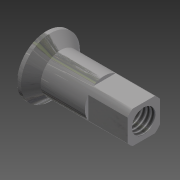
# Autodesk Inventor part: Nypel_szprychy
Saved by Autodesk Inventor 2015 (Build 190159000, 159)
## iProperties
Created: 2015-11-24
Part Number: Nypel_szprychy
Material: Stal nierdzewna
Document SubType Name: Modeling
Designer: graaapsik
Density: 8.08 g/cm^3
Appearance: Częściowo polerowany
Author: graaapsik
Autodesk Inventor part; units mm, degrees
ref_plane "YZ Plane" through (0, 0, 0) normal (1, 0, 0) x (0, 1, 0)
ref_plane "XZ Plane" through (0, 0, 0) normal (0, 1, 0) x (-1, 0, 0)
ref_plane "XY Plane" through (0, 0, 0) normal (0, 0, 1) x (1, 0, 0)
sketch "Szkic1" plane through (0, 0, 0) normal (0, 0, 1) x (1, 0, 0)
  line L0 (9.9, 0) -> (9.9, 2)
  line L1 (9.9, 2) -> (1.4, 2)
  line L2 (1.4, 2) -> (0.4, 3)
  line L3 (0.4, 3) -> (0, 3)
  arc A0 (0, 3) -> (-1.4487, 0) centre (8.1549, -2.7877) ccw
  line L4 (-1.1, 1) -> (9.9, 1) construction
  line L5 (-1.4487, 0) -> (0, 0)
  line L6 (9.9, 0) -> (0, 0)
  dimension "d1" = 11
  dimension "d2" = 1.1
  dimension "d3" = 10
  dimension "d9" = 2.5
  dimension "d10" = 45
  dimension "d11" = 1
  dimension "d12" = 3
  constraints: 14 end point, 5 point on circle, 3 horizontal, 1 centre point, 1 coincident, 1 collinear, 1 midpoint, 1 parallel, 1 vertical, 1 vertical alignment
  measures "d1" distance from line of L0 L4.start
  measures "d2" horizontal distance of L3.end L4.start
  measures "d3" radius of A0
  measures "d9" horizontal distance of L1.end L4.start
  measures "d10" angle of L4 L2
  measures "d11" distance between parallel lines of L6 L4
  measures "d12" distance between parallel lines of L3 L6
revolve "Obrót1" add sketch "Szkic1" angle 360 about axis through (9.9, 0, 0) along (-1, 0, 0)
sketch "Szkic2" plane through (9.9, 0, 0) normal (1, 0, 0) x (0, 0, -1)
  circle A0 centre (0, 0) radius 2 projected
  line L0 (-1.1303, -1.65) -> (1.1303, -1.65)
  line L1 (1.65, -1.1303) -> (1.65, 1.1303)
  line L2 (1.1303, 1.65) -> (-1.1303, 1.65)
  line L3 (-1.65, 1.1303) -> (-1.65, -1.1303)
  line L4 (-1.65, -1.65) -> (1.65, 1.65) construction
  line L5 (1.65, -1.65) -> (-1.65, 1.65) construction
  dimension "d14" = 3.3
  dimension "d15" = 3.3
  constraints: 12 end point, 2 midpoint, 2 parallel, 1 horizontal, 1 perpendicular, 9 other
  measures "d14" distance of L5.end L4.end
  measures "d15" distance of L5.start L4.end
extrude "Wyciągnięcie proste2" cut sketch "Szkic2" against normal blind 4 contours A0 L1 | L2 A0 | A0 L0 | L3 A0
sketch "Szkic3" plane through (9.9, -1.1303, -1.65) normal (1, 0, 0) x (0, 0, -1)
  line L0 (-2.7803, -0.5197) -> (-0.5197, -0.5197) projected
  arc A0 (-0.5197, -0.5197) -> (0, 0) centre (-1.65, 1.1303) ccw projected
  line L1 (0, 0) -> (0, 2.2605) projected
  arc A1 (0, 2.2605) -> (-0.5197, 2.7803) centre (-1.65, 1.1303) ccw projected
  line L2 (-0.5197, 2.7803) -> (-2.7803, 2.7803) projected
  arc A2 (-2.7803, 2.7803) -> (-3.3, 2.2605) centre (-1.65, 1.1303) ccw projected
  line L3 (-3.3, 2.2605) -> (-3.3, 0) projected
  arc A3 (-3.3, 0) -> (-2.7803, -0.5197) centre (-1.65, 1.1303) ccw projected
  constraints: 1 coincident
hole "Otwór1" at (9.9, 0, 0) direction (-1, 0, 0) diameter 1.8 end through all counterbore diameter 2.4 counterbore depth 2.5
chamfer "Faza1" distance 0.25 angle 45 1 edges at (7.4, 0, 0.9)
chamfer "Faza2" distance 0.25 angle 45 2 edges at (-1.1403, -0.6363, 0.6365) (-1.1403, 0.6364, -0.6364)
sketch "Szkic5" plane through (0, 0, 0) normal (0, 1, 0) x (-1, 0, 0)
  line L0 (0, 3) -> (0, -3) construction
  line L1 (1.0546, -0.55) -> (-0.0454, -0.55)
  line L2 (-0.0454, -0.55) -> (-0.0454, 0.55)
  line L3 (-0.0454, 0.55) -> (1.0546, 0.55)
  line L4 (1.0546, 0.55) -> (1.0546, -0.55)
  line L5 (1.0546, -0.55) -> (-0.0454, 0.55) construction
  line L6 (-0.0454, -0.55) -> (1.0546, 0.55) construction
  point P0 (0, 0)
  point P1 (0.5046, 0)
  dimension "d33" = 1.1
  dimension "d34" = 1.1
  constraints: 12 end point, 2 midpoint, 2 parallel, 2 perpendicular
  measures "d33" distance of L3.end L1.start
  measures "d34" distance of L2.end L3.end
extrude "Wyciągnięcie proste3" cut sketch "Szkic5" along normal through all both and the other way through all
thread "Gwint1" size "M2.5x0.45" class "6H" standard "ANSI Metric M Profile" full length
